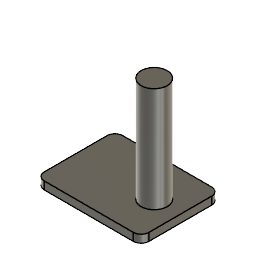
Raupen_Halterung (Autodesk Fusion 360 design; units mm, degrees)
part number: 2026-05-31-14-33-19-862
Autodesk Fusion 360 part; units mm, degrees
sketch "Skizze1" plane through (0, 0, 0) normal (0, 0, 1) x (1, 0, 0)
  line L0 (0, 10) -> (40, 10)
  line L1 (40, 10) -> (40, -20)
  line L2 (40, -20) -> (0, -20)
  line L3 (0, -20) -> (0, 10)
  dimension "d1" = 40
  dimension "d2" = 30
  constraint horizontal L0
  constraint vertical L1
  constraint horizontal L2
  constraint vertical L3
  measures "d1" distance of L0.start L0.end
  measures "d2" distance of L0.end L1.end
extrude "Extrusion1" add sketch "Skizze1" along normal blind 3
fillet "Abrundung1" radius 3 4 edges at (0, -20, 1.5) (40, -20, 1.5) (40, 10, 1.5) (0, 10, 1.5)
sketch "Skizze2" plane through (0, 0, 3) normal (0, 0, 1) x (-1, 0, 0)
  arc A0 (-3, -10) -> (0, -7) centre (-3, -7) ccw
  line L0 (0, -7) -> (0, 17)
  arc A1 (0, 17) -> (-3, 20) centre (-3, 17) ccw
  line L1 (-3, 20) -> (-37, 20)
  arc A2 (-37, 20) -> (-40, 17) centre (-37, 17) ccw
  line L2 (-40, 17) -> (-40, -7)
  arc A3 (-40, -7) -> (-37, -10) centre (-37, -7) ccw
  line L3 (-37, -10) -> (-3, -10)
  circle A4 centre (-30, 5) radius 5
extrude "Extrusion2" add sketch "Skizze2" along normal blind 40 contours A4
